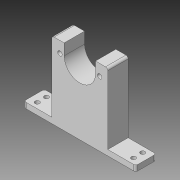
# Autodesk Inventor part: STEPPER MOTOR MOUNT
Saved by Autodesk Inventor 2017 (Build 210142000, 142)
## iProperties
Created: 2017-03-25
Part Number: STEPPER MOTOR MOUNT
Material: Generic
Document SubType Name: Modeling
Designer: Muchen
Density: 1 g/cm^3
Appearance: Default
Mass: 53.1535 g
Surface Area: 131.208 cm^2
Volume: 53.1535 cm^3
Author: Muchen
Autodesk Inventor part; units mm, degrees
ref_plane "YZ Plane" through (0, 0, 0) normal (1, 0, 0) x (0, 1, 0)
ref_plane "XZ Plane" through (0, 0, 0) normal (0, 1, 0) x (-1, 0, 0)
ref_plane "XY Plane" through (0, 0, 0) normal (0, 0, 1) x (1, 0, 0)
sketch "Sketch1" plane through (0, 0, 0) normal (0, 0, 1) x (1, 0, 0)
  line L0 (0, 65.5357) -> (0, 44) construction
  line L1 (0, 0) -> (50, 0)
  line L2 (50, 0) -> (50, 5)
  line L3 (50, 5) -> (25, 5)
  line L4 (25, 5) -> (25, 68)
  line L5 (25, 68) -> (14, 68)
  line L6 (14, 68) -> (14, 58)
  arc A0 (0, 44) -> (14, 58) centre (0, 58) ccw
  circle A1 centre (17.75, 58) radius 2
  line L7 (0, 44) -> (0, 0)
  point P0 (0, 50)
  dimension "d0" = 5
  dimension "d1" = 50
  dimension "d2" = 25
  dimension "d4" = 14
  dimension "d5" = 4
  dimension "d6" = 17.75
  dimension "d7" = 10
  dimension "d22" = 50
  dimension "d23" = 6
  constraints: 16 end point, 6 perpendicular, 2 centre point, 2 line through centre, 2 point on circle, 2 vertical, 1 horizontal alignment, 1 point on line, 1 tangent
  measures "d0" distance of L1.end L2.end
  measures "d1" distance between parallel lines of L2 L0
  measures "d2" distance between parallel lines of L0 L4
  measures "d4" distance between parallel lines of L6 L0
  measures "d5" diameter of A1
  measures "d6" distance from line of A1.centre L0
  measures "d7" distance from line of L5 A0.centre
  measures "d22" distance from line of L1 point (0, 50)
  measures "d23" distance of point (0, 50) L0.end
extrude "Extrusion1" add sketch "Sketch1" along normal blind 18.2
mirror "Mirror1" about plane through (0, 0, 0) normal (1, 0, 0) of "Extrusion1"
sketch "Sketch2" plane through (50, 0, 0) normal (0, -1, 0) x (1, 0, 0)
  line L0 (-75, 0) -> (-75, 18.2) projected
  line L1 (-25, 0) -> (-25, 18.2) projected
  line L2 (-100, 0) -> (-100, 18.2) projected
  line L3 (0, 0) -> (0, 18.2) projected
  line L4 (0, 18.2) -> (-100, 18.2) projected
  line L5 (-100, 0) -> (0, 0) projected
  point P0 (-50, 0)
  point P1 (-93, 13.2)
  point P2 (-93, 5)
  point P3 (-7, 5)
  point P4 (-7, 13.2)
  dimension "d10" = 7
  dimension "d11" = 7
  dimension "d12" = 5
  dimension "d13" = 5
  constraints: 2 horizontal alignment, 2 vertical alignment
  measures "d10" distance from line of L3 point (-7, 13.2)
  measures "d11" distance from line of L2 point (-93, 13.2)
  measures "d12" distance from line of L4 point (-93, 13.2)
  measures "d13" distance from line of L5 point (-93, 5)
hole "Hole1" at (-43, 0, 13.2) at (-43, 0, 5) at (43, 0, 5) at (43, 0, 13.2) direction (0, 1, 0) diameter 4 end through all
fillet "Fillet1" radius 2 6 edges at (-50, 2.5, 18.2) (-50, 2.5, 0) (50, 2.5, 0) (50, 2.5, 18.2) (25, 68, 9.1) (-25, 68, 9.1)
body "Solid1"
